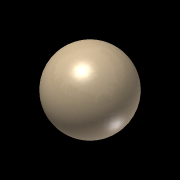
# Autodesk Inventor part: Ball
Saved by Autodesk Inventor 2014 SP1 (Build 180222100, 222)
## iProperties
Created: 2014-04-13
Part Number: Ball
Material: Polyethylene, High Density
Document SubType Name: Modeling
Designer: Rauhul Varma
Density: 0.952 g/cm^3
Appearance: Smooth - Off-White
Mass: 0.127631 g
Surface Area: 1.26677 cm^2
Volume: 0.134066 cm^3
Author: Rauhul Varma
Autodesk Inventor part; units mm, degrees
ref_plane "YZ Plane" through (0, 0, 0) normal (1, 0, 0) x (0, 1, 0)
ref_plane "XZ Plane" through (0, 0, 0) normal (0, 1, 0) x (-1, 0, 0)
ref_plane "XY Plane" through (0, 0, 0) normal (0, 0, 1) x (1, 0, 0)
sketch "Sketch2" plane through (0, 0, 0) normal (0, 0, 1) x (1, 0, 0)
  circle A0 centre (0, 0) radius 3.175
  line L0 (-0.7646, 3.0816) -> (0.7646, -3.0816)
  dimension "d0" = 6.35
  constraints: 2 end point, 2 point on circle, 1 centre point, 1 coincident, 1 midpoint
  measures "d0" diameter of A0
revolve "Revolution1" add sketch "Sketch2" angle 360 about axis through (-0.7646, 3.0816, 0) along (0.2408182, -0.9705702, 0) picked at (-1.5425, 0.004) contours L0 A0
body "Solid1"
